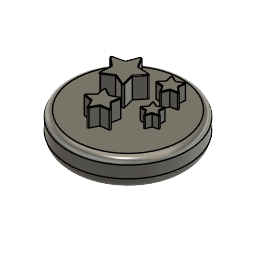
PIN5 (Autodesk Fusion 360 design; units mm, degrees)
Autodesk Fusion 360 part; units mm, degrees
sketch "Sketch1" plane through (0, 0, 0) normal (0, 1, 0) x (1, 0, 0)
  line L0 (0, 0) -> (5, 0)
  line L1 (5, 0) -> (5, 5)
  line L2 (5, 5) -> (0, 5)
  line L3 (0, 5) -> (0, 0)
  dimension "d1" = 5
  dimension "d2" = 5
  constraint horizontal L0
  constraint vertical L1
  constraint horizontal L2
  constraint vertical L3
  constraint coincident L0.start L3.end
  measures "d1" distance of L0.start L0.end
  measures "d2" distance of L0.start L2.end
extrude "Extrude1" add sketch "Sketch1" along normal blind 3.8
sketch "Sketch2" plane through (0, 3.8, 0) normal (0, 1, 0) x (-1, 0, 0)
  line L0 (0, -5) -> (0, 0)
  line L1 (0, 0) -> (-5, 0)
  line L2 (-5, 0) -> (-5, -5)
  line L3 (-5, -5) -> (0, -5)
  circle A0 centre (-2.5, -2.5) radius 10
  dimension "d5" = 20
  measures "d5" diameter of A0
extrude "Extrude2" add sketch "Sketch2" along normal blind 5 contours L0 L1 L2 L3 | A0
fillet "Fillet1" radius 1 1 edges at (11.8233, 8.8, -6.1162)
fillet "Fillet1" radius 2 1 edges at (11.8233, 3.8, -6.1162)
sketch "Sketch4" plane through (0, 8.8, 0) normal (0, 1, 0) x (-1, 0, 0)
  circle A0 centre (-2.5, -2.5) radius 9
  line L0 (1.8228, -4.0272) -> (0.1014, -3.009)
  line L1 (0.1014, -3.009) -> (-1.3989, -4.3316)
  line L2 (-1.3989, -4.3316) -> (-0.6047, -6.1671)
  line L3 (-0.6047, -6.1671) -> (1.3864, -5.979)
  line L4 (1.3864, -5.979) -> (1.8228, -4.0272)
  line L5 (0.7243, -7.6981) -> (1.3864, -5.979)
  line L6 (-0.6047, -6.1671) -> (0.3678, -7.7318)
  arc A1 (0.3678, -7.7318) -> (0.7243, -7.6981) centre (0.5376, -7.6262) ccw
  line L7 (1.3864, -5.979) -> (3.1751, -5.5376)
  arc A2 (3.1751, -5.5376) -> (3.2532, -5.1882) centre (3.1271, -5.3435) ccw
  line L8 (3.2532, -5.1882) -> (1.8228, -4.0272)
  line L9 (1.8228, -4.0272) -> (1.9558, -2.1897)
  arc A3 (1.9558, -2.1897) -> (1.6476, -2.0074) centre (1.7563, -2.1753) ccw
  line L10 (1.6476, -2.0074) -> (0.1014, -3.009)
  line L11 (0.1014, -3.009) -> (-1.6051, -2.3147)
  arc A4 (-1.6051, -2.3147) -> (-1.8737, -2.5515) centre (-1.6804, -2.5) ccw
  line L12 (-1.8737, -2.5515) -> (-1.3989, -4.3316)
  line L13 (-1.3989, -4.3316) -> (-2.5865, -5.7399)
  arc A5 (-2.5865, -5.7399) -> (-2.4443, -6.0686) centre (-2.4336, -5.8689) ccw
  line L14 (-2.4443, -6.0686) -> (-0.6047, -6.1671)
  line L15 (-7.2222, -3.0294) -> (-6.3527, -3.5233)
  line L16 (-6.3527, -3.5233) -> (-5.4936, -3.8555)
  arc A6 (-7.2727, -3.9491) -> (-7.117, -4.0376) centre (-7.1728, -3.9546) ccw
  line L17 (-5.3614, -3.7348) -> (-5.6143, -2.8491)
  arc A7 (-7.9114, -2.2861) -> (-7.9474, -2.4614) centre (-7.8858, -2.3827) ccw
  line L18 (-5.6143, -2.8491) -> (-6.0273, -1.9384)
  line L19 (-6.0273, -1.9384) -> (-6.5271, -1.1646)
  arc A8 (-6.5271, -1.1646) -> (-6.7051, -1.1846) centre (-6.6111, -1.2189) ccw
  line L20 (-5.1068, -1.9716) -> (-6.0273, -1.9384)
  line L21 (-7.117, -4.0376) -> (-6.3527, -3.5233)
  arc A9 (-5.4936, -3.8555) -> (-5.3614, -3.7348) centre (-5.4575, -3.7623) ccw
  line L22 (-7.9474, -2.4614) -> (-7.2222, -3.0294)
  line L23 (-7.0211, -2.0498) -> (-7.9114, -2.2861)
  arc A10 (-5.0328, -2.1346) -> (-5.1068, -1.9716) centre (-5.1104, -2.0715) ccw
  line L24 (-5.6143, -2.8491) -> (-5.0328, -2.1346)
  line L25 (-7.2222, -3.0294) -> (-7.2727, -3.9491)
  line L26 (-6.7051, -1.1846) -> (-7.0211, -2.0498)
  line L27 (-6.0273, -1.9384) -> (-7.0211, -2.0498)
  line L28 (-7.0211, -2.0498) -> (-7.2222, -3.0294)
  line L29 (-6.3527, -3.5233) -> (-5.6143, -2.8491)
  line L30 (-0.9784, 2.1936) -> (-2.4783, 2.2093)
  line L31 (-1.7526, -0.1067) -> (-0.5342, -0.7583)
  line L32 (-1.8496, 3.4397) -> (-2.4783, 2.2093)
  line L33 (-2.4783, 2.2093) -> (-3.847, 2.0203)
  arc A11 (-1.5811, 3.4369) -> (-1.8496, 3.4397) centre (-1.7161, 3.3714) ccw
  line L34 (-0.5299, 0.7622) -> (0.4663, 1.7196)
  arc A12 (-3.2, -0.5724) -> (-2.9844, -0.7326) centre (-3.0524, -0.5988) ccw
  arc A13 (-3.847, 2.0203) -> (-3.9327, 1.7658) centre (-3.8265, 1.8718) ccw
  line L35 (-1.7526, -0.1067) -> (-0.5299, 0.7622)
  line L36 (-2.9844, -0.7326) -> (-1.7526, -0.1067)
  line L37 (-3.9327, 1.7658) -> (-2.9568, 0.7877)
  arc A14 (-0.5342, -0.7583) -> (-0.3153, -0.6028) centre (-0.4635, -0.626) ccw
  line L38 (-0.3153, -0.6028) -> (-0.5299, 0.7622)
  line L39 (-2.4783, 2.2093) -> (-2.9568, 0.7877)
  arc A15 (0.4663, 1.7196) -> (0.386, 1.9758) centre (0.3624, 1.8277) ccw
  line L40 (0.386, 1.9758) -> (-0.9784, 2.1936)
  line L41 (-0.9784, 2.1936) -> (-1.5811, 3.4369)
  line L42 (-0.5299, 0.7622) -> (-0.9784, 2.1936)
  line L43 (-2.9568, 0.7877) -> (-3.2, -0.5724)
  line L44 (-2.9568, 0.7877) -> (-1.7526, -0.1067)
  line L45 (-4.8449, -8.2445) -> (-3.8284, -8.6788)
  line L46 (-4.3882, -6.3573) -> (-5.5847, -6.4493)
  arc A16 (-6.6623, -6.6954) -> (-6.7129, -6.9042) centre (-6.6356, -6.8123) ccw
  arc A17 (-5.9659, -8.7166) -> (-5.7829, -8.8292) centre (-5.8464, -8.7273) ccw
  arc A18 (-3.8284, -8.6788) -> (-3.6648, -8.5396) centre (-3.7813, -8.5685) ccw
  line L47 (-5.1695, -5.4249) -> (-5.5847, -6.4493)
  line L48 (-3.6648, -8.5396) -> (-3.931, -7.4668)
  arc A19 (-3.2038, -6.6343) -> (-3.2857, -6.4357) centre (-3.2942, -6.5554) ccw
  arc A20 (-4.9552, -5.4084) -> (-5.1695, -5.4249) centre (-5.0582, -5.47) ccw
  line L49 (-5.5847, -6.4493) -> (-6.6623, -6.6954)
  line L50 (-4.3882, -6.3573) -> (-4.9552, -5.4084)
  line L51 (-5.7829, -8.8292) -> (-4.8449, -8.2445)
  line L52 (-5.8669, -7.6157) -> (-5.9659, -8.7166)
  line L53 (-5.5847, -6.4493) -> (-5.8669, -7.6157)
  line L54 (-4.8449, -8.2445) -> (-3.931, -7.4668)
  line L55 (-3.931, -7.4668) -> (-4.3882, -6.3573)
  line L56 (-5.8669, -7.6157) -> (-4.8449, -8.2445)
  line L57 (-3.2857, -6.4357) -> (-4.3882, -6.3573)
  line L58 (-6.7129, -6.9042) -> (-5.8669, -7.6157)
  line L59 (-3.931, -7.4668) -> (-3.2038, -6.6343)
  point P0 (0.2614, -4.7028)
  point P1 (-7.3816, -0.7984)
  point P2 (-6.4475, -2.678)
  point P3 (-4.3588, 1.5644)
  point P4 (-1.7392, 1.1692)
  point P5 (-7.0384, -7.0944)
  point P6 (-4.9231, -7.2267)
  dimension "d12" = 2
  dimension "d14" = 0.2
  dimension "d16" = 360
  dimension "d18" = 360
  dimension "d22" = 360
  dimension "d26" = 360
  constraint tangent L5 A1
  constraint tangent L6 A1
  constraint tangent A6 L21
  constraint tangent A6 L25
  constraint tangent A14 L38
  constraint tangent L31 A14
  constraint tangent A18 L48
  constraint tangent L45 A18
  measures "d12" distance of L0.start L3.end
  measures "d14" radius of A1
extrude "Extrude3" add sketch "Sketch4" along normal blind 3.5 contours L0 L1 L2 L3 L4 | L4 L7 A2 L8 | L0 L9 A3 L10 | L1 L11 A4 L12 | L3 L5 L6 A1 | L2 L13 A5 L14
extrude "Extrude4" add sketch "Sketch4" along normal blind 3 contours L30 L35 L39 L42 L44 | L30 L32 A11 L41 | L34 A15 L40 L42 | L33 A13 L37 L39 | L31 L35 A14 L38 | A12 L36 L43 L44
extrude "Extrude5" add sketch "Sketch4" along normal blind 2 contours L15 L18 L27 L28 L29 | L15 A6 L21 L25 | A7 L22 L23 L28 | L16 L17 A9 L29 | L19 A8 L26 L27 | L18 L20 A10 L24
extrude "Extrude6" add sketch "Sketch4" along normal blind 2.5 contours L45 A18 L48 L54 | L46 L53 L54 L55 L56 | A17 L51 L52 L56 | A19 L55 L57 L59 | A16 L49 L53 L58 | L46 L47 A20 L50
fillet "Fillet2" radius 0.1 60 edges at (-1.8893, 12.3, -3.1084) (-1.8581, 12.3, -2.0031) (-0.8745, 12.3, -2.5082) (0.7518, 12.3, -2.6619) (1.8127, 12.3, -2.35) (1.6363, 12.3, -3.4416) (1.9927, 12.3, -5.0358) (2.6172, 12.3, -5.9483) (1.5245, 12.3, -6.1179) (0.1185, 12.3, -6.9495) (-0.5565, 12.3, -7.8253) (-1.0554, 12.3, -6.8385) (-2.2808, 12.3, -5.7583) (-3.3223, 12.3, -5.3871) (-2.538, 12.3, -4.6077) (3.1627, 11.8, 2.1148) (3.9687, 11.8, 1.9196) (3.4448, 11.8, 1.2767) (1.1434, 11.8, -0.4325) (0.3766, 11.8, -0.7483) (0.4226, 11.8, 0.0797) (3.0784, 11.8, 0.1076) (3.1418, 11.8, -0.7193) (2.3685, 11.8, -0.4196) (0.0318, 11.8, 1.2409) (-0.5055, 11.8, 1.8726) (0.2962, 11.8, 2.0847) (1.2798, 11.8, 2.8152) (1.7145, 11.8, 3.5214) (2.164, 11.8, 2.8245) (5.3235, 10.8, -2.4919) (5.0193, 10.8, -2.0302) (5.5671, 10.8, -1.955) (5.9232, 10.8, -3.6894) (5.3901, 10.8, -3.8361) (5.4878, 10.8, -3.2919) (7.2474, 10.8, -3.4892) (7.2222, 10.8, -4.0415) (6.7349, 10.8, -3.7805) (7.4663, 10.8, -2.1679) (7.9837, 10.8, -2.3626) (7.5848, 10.8, -2.7454) (6.2772, 10.8, -1.5515) (6.6223, 10.8, -1.1195) (6.8631, 10.8, -1.6172) (4.6717, 11.3, -5.8829) (5.0674, 11.3, -5.3504) (5.3771, 11.3, -5.9371) (3.5674, 11.3, -7.0505) (3.1832, 11.3, -6.5096) (3.8369, 11.3, -6.3965) (4.3366, 11.3, -8.4617) (3.7035, 11.3, -8.6599) (3.7979, 11.3, -8.0032) (5.9164, 11.3, -8.1661) (5.9093, 11.3, -8.8295) (5.3139, 11.3, -8.5368) (6.1235, 11.3, -6.5723) (6.7522, 11.3, -6.7841) (6.2899, 11.3, -7.2599)
chamfer "Chamfer1" distance 1 angle 45 4 edges at (0, 0, -2.5) (2.5, 0, -5) (5, 0, -2.5) (2.5, 0, 0)
